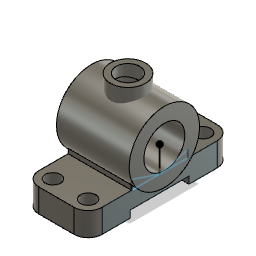
drawing_15 v1 (Autodesk Fusion 360 design; units mm, degrees)
Autodesk Fusion 360 part; units mm, degrees
note: some values were not read from the file. Set by a fixed rule: which sketch regions a step uses.
sketch "Sketch1" plane through (0, 0, 0) normal (0, 1, 0) x (1, 0, 0)
  line L0 (17, -5) -> (47, -5)
  line L1 (59, -17) -> (59, -115)
  line L2 (47, -127) -> (17, -127)
  line L3 (5, -115) -> (5, -17)
  arc A0 (17, -5) -> (5, -17) centre (17, -17) ccw
  arc A1 (59, -17) -> (47, -5) centre (47, -17) ccw
  arc A2 (5, -115) -> (17, -127) centre (17, -115) ccw
  arc A3 (47, -127) -> (59, -115) centre (47, -115) ccw
  circle A4 centre (17, -115) radius 6.5
  circle A5 centre (17, -17) radius 6.5
  circle A6 centre (47, -17) radius 6.5
  circle A7 centre (47, -115) radius 6.5
  point P0 (5, -5)
  point P1 (59, -5)
  point P2 (5, -127)
  dimension "d1" = 54
  dimension "d2" = 122
  dimension "d3" = 12
  dimension "d4" = 12
  dimension "d5" = 12
  dimension "d6" = 12
  dimension "d7" = 13
  dimension "d8" = 13
  dimension "d9" = 13
  dimension "d10" = 13
  constraint horizontal L0
  constraint vertical L1
  constraint horizontal L2
  constraint vertical L3
  constraint coincident P0 L0
  constraint coincident P0 L3
  constraint tangent L0 A0
  constraint tangent L3 A0
  constraint coincident P1 L0
  constraint coincident P1 L1
  constraint tangent L0 A1
  constraint tangent L1 A1
  constraint coincident P2 L2
  constraint coincident P2 L3
  constraint tangent L2 A2
  constraint tangent L3 A2
  constraint tangent L1 A3
  constraint tangent L2 A3
  constraint concentric A2 A4
  constraint concentric A0 A5
  constraint concentric A1 A6
  constraint concentric A3 A7
  measures "d1" distance of P0 P1
  measures "d2" distance of P0 P2
  measures "d3" radius of A0
  measures "d4" radius of A1
  measures "d5" radius of A2
  measures "d6" radius of A3
  measures "d7" diameter of A4
  measures "d8" diameter of A5
  measures "d9" diameter of A6
  measures "d10" diameter of A7
extrude "Extrude1" add sketch "Sketch1" along normal blind 20 makes body 1
sketch "Sketch2" plane through (59, 0, 0) normal (1, 0, 0) x (0, 0, -1)
  line L0 (-115, 0) -> (-17, 0)
  line L1 (-17, 0) -> (-17, 20)
  line L2 (-17, 20) -> (-115, 20)
  line L3 (-115, 20) -> (-115, 0)
  line L4 (-127, 0) -> (-66, 0)
  line L5 (-66, 0) -> (-41, 0)
  line L6 (-41, 0) -> (-91, 0)
  line L7 (-91, 0) -> (-91, 6)
  line L8 (-91, 6) -> (-41, 6)
  line L9 (-41, 6) -> (-41, 0)
  dimension "d13" = 61
  dimension "d14" = 25
  dimension "d15" = 50
  dimension "d16" = 6
  constraint parallel L0 L4
  constraint parallel L0 L5
  constraint horizontal L6
  constraint vertical L7
  constraint horizontal L8
  constraint vertical L9
  measures "d13" distance of L4.start L4.end
  measures "d14" distance of L4.end L5.end
  measures "d15" distance of L5.end L6.end
  measures "d16" distance of L5.end L8.end
extrude "Extrude2" cut sketch "Sketch2" against normal blind 175 contours L0 L4 L5 L6 L7 L8 L9 bodies 1
sketch "Sketch3" plane through (0, 0, 0) normal (1, 0, 0) x (0, 0, -1)
sketch "Sketch4" plane through (59, 0, 0) normal (1, 0, 0) x (0, 0, -1)
  line L0 (-41, 6) -> (-41, 0)
  line L1 (-41, 0) -> (-17, 0)
  line L2 (-17, 0) -> (-17, 20)
  line L3 (-17, 20) -> (-115, 20)
  line L4 (-115, 20) -> (-115, 0)
  line L5 (-115, 0) -> (-91, 0)
  line L6 (-91, 0) -> (-91, 6)
  line L7 (-91, 6) -> (-41, 6)
  line L8 (-5, 20) -> (-66, 20)
  line L9 (-66, 20) -> (-66, 32)
  line L10 (-66, 32) -> (-66, 42)
  circle A0 centre (-66, 42) radius 30
  dimension "d19" = 12
  dimension "d20" = 10
  dimension "d21" = 60
  constraint midpoint L3 L8.end
  constraint perpendicular L4 L8
  constraint perpendicular L8 L9
  constraint parallel L9 L10
  constraint coincident L10.end A0.centre
  measures "d19" distance of L8.end L9.end
  measures "d20" distance of L9.end L10.end
  measures "d21" diameter of A0
extrude "Extrude3" add sketch "Sketch4" along normal blind 4 contours L3 L8 A0 | L3 L8 A0 bodies 1
extrude "Extrude4" cut sketch "Sketch4" against normal blind 55 contours L3 L8 A0 | L3 L8 A0 bodies 1
extrude "Extrude5" add 1 faces at (59, 51.0141, 63.6991) along direction (-1, 0, 0) blind 58 on bodies 1 bodies 1
hole "Hole1" at (63, 42, 66) direction (-1, 0, 0) diameter 35 depth 48 tip angle 180 bodies 1
ref_plane "WorkPlane1" through (32, 76, 66) normal (0, -1, 0) x (0, 0, 1)
sketch "Sketch5" plane through (32, 76, 66) normal (0, -1, 0) x (1, 0, 0)
  circle A0 centre (0, 0) radius 15
  dimension "d32" = 30
  constraint coincident A0.centre origin
  measures "d32" diameter of A0
sketch "Sketch6" plane through (32, 76, 66) normal (0, -1, 0) x (1, 0, 0)
extrude "Extrude6" add sketch "Sketch5" against normal blind 5 separate body makes body 2
move_face "OffsetFaces1" offset 10 1 faces at (29.3337, 76, 72.5491) on bodies 2
hole "Hole2" at (32, 81, 66) direction (0, -1, 0) diameter 20 depth 100 tip angle 180 bodies 1 2
sketch "Sketch7" plane through (59, 0, 0) normal (1, 0, 0) x (0, 0, -1)
  arc A0 (-86.3961, 20) -> (-45.6039, 20) centre (-66, 42) ccw
  line L0 (-86.3961, 20) -> (-115, 20)
  line L1 (-115, 20) -> (-115, 0)
  line L2 (-115, 0) -> (-91, 0)
  line L3 (-91, 0) -> (-91, 6)
  line L4 (-91, 6) -> (-41, 6)
  line L5 (-41, 6) -> (-41, 0)
  line L6 (-41, 0) -> (-17, 0)
  line L7 (-17, 0) -> (-17, 20)
  line L8 (-17, 20) -> (-45.6039, 20)
  line L9 (-66, 42) -> (-66, 20)
  line L10 (-66, 20) -> (-90, 20)
  line L11 (-90, 20) -> (-90, 28)
  line L12 (-90, 28) -> (-66, 20)
  line L13 (-66, 20) -> (-42, 20)
  line L14 (-42, 20) -> (-42, 26)
  line L15 (-42, 26) -> (-66, 20)
  dimension "d39" = 24
  dimension "d40" = 24
  constraint coincident A0.centre L9.start
  constraint vertical L9
  constraint perpendicular L9 L10
  constraint perpendicular L0 L11
  constraint perpendicular L9 L13
  constraint perpendicular L8 L14
  measures "d39" distance of L9.end L10.end
  measures "d40" distance of L9.end L13.end
extrude "Extrude8" add sketch "Sketch7" against normal blind 54 contours L8 L13 L14 L15 bodies 1
hole "Hole3" at (1, 42, 66) direction (1, 0, 0) diameter 20 depth 100 tip angle 180 bodies 1
extrude "Extrude7" add sketch "Sketch7" against normal blind 54 contours L0 L10 L11 L12 bodies 1
